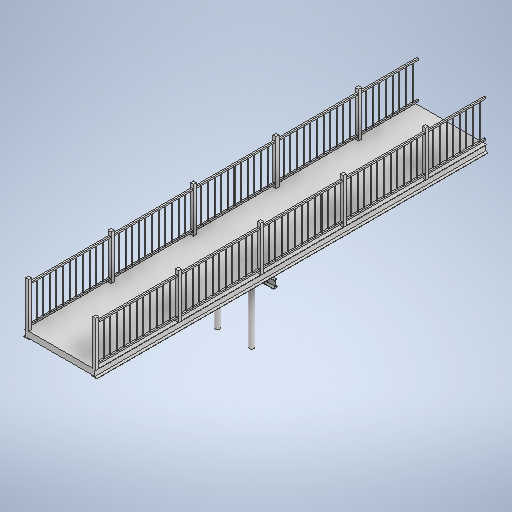
# Autodesk Inventor part: Bridge for Jude
Saved by Autodesk Inventor 2025 (Build 290162000, 162)
## iProperties
Created: 2024-06-25
Part Number: Bridge for Jude
Material: Generic
Document SubType Name: Modeling
Designer: track
Density: 1 g/cm^3
Appearance: Default
Author: track
Autodesk Inventor part; units mm, degrees
ref_plane "YZ Plane" through (0, 0, 0) normal (1, 0, 0) x (0, 1, 0)
ref_plane "XZ Plane" through (0, 0, 0) normal (0, 1, 0) x (-1, 0, 0)
ref_plane "XY Plane" through (0, 0, 0) normal (0, 0, 1) x (1, 0, 0)
sketch "Sketch4" plane through (0, 0, 0) normal (0, 0, 1) x (1, 0, 0)
  line L0 (838.2, -76.2) -> (-838.2, -76.2)
  line L1 (-838.2, -76.2) -> (-838.2, 76.2)
  line L2 (-838.2, 76.2) -> (838.2, 76.2)
  line L3 (838.2, 76.2) -> (838.2, -76.2)
  line L4 (838.2, -76.2) -> (-838.2, 76.2) construction
  line L5 (-838.2, -76.2) -> (838.2, 76.2) construction
  point P0 (0, 0)
  dimension "d8" = 1676.4
  dimension "d9" = 152.4
  constraints: 12 end point, 2 midpoint, 2 parallel, 1 horizontal, 1 perpendicular
  measures "d8" distance of L1.end L2.end
  measures "d9" distance of L0.end L1.end
extrude "Extrusion2" add sketch "Sketch4" against normal blind 9753.6
sketch "Sketch5" plane through (0, 0, 0) normal (0, 0, 1) x (1, 0, 0)
  line L0 (787.4, -101.6) -> (914.4, -101.6)
  line L1 (863.6, -76.2) -> (863.6, 50.8)
  line L2 (838.2, -76.2) -> (838.2, 50.8)
  line L3 (-838.2, 76.2) -> (838.2, 76.2) projected
  line L4 (889, 76.2) -> (812.8, 76.2)
  line L5 (-838.2, -76.2) -> (838.2, -76.2) projected
  line L6 (787.4, -101.6) -> (787.4, -95.25)
  line L7 (787.4, -95.25) -> (838.2, -76.2)
  line L8 (914.4, -101.6) -> (914.4, -95.25)
  line L9 (914.4, -95.25) -> (863.6, -76.2)
  line L10 (889, 76.2) -> (889, 66.675)
  line L11 (889, 66.675) -> (863.6, 50.8)
  line L12 (838.2, -76.2) -> (838.2, 76.2) projected
  line L13 (850.9, -101.6) -> (850.9, -34.364)
  line L14 (838.2, 50.8) -> (863.6, 50.8)
  line L15 (0, -76.2) -> (0, 76.2)
  line L16 (-787.4, -101.6) -> (-914.4, -101.6)
  line L17 (-863.6, -76.2) -> (-863.6, 50.8)
  line L18 (-838.2, -76.2) -> (-838.2, 50.8)
  line L19 (-889, 76.2) -> (-812.8, 76.2)
  line L20 (-787.4, -101.6) -> (-787.4, -95.25)
  line L21 (-787.4, -95.25) -> (-838.2, -76.2)
  line L22 (-914.4, -95.25) -> (-863.6, -76.2)
  line L23 (-889, 76.2) -> (-889, 66.675)
  line L24 (-889, 66.675) -> (-863.6, 50.8)
  line L25 (-787.4, -101.6) -> (-787.4, -95.25)
  line L26 (-914.4, -101.6) -> (-914.4, -95.25)
  line L27 (838.2, 50.8) -> (812.8, 66.675)
  line L28 (812.8, 66.675) -> (812.8, 76.2)
  line L29 (-838.2, 50.8) -> (-812.8, 66.675)
  line L30 (-812.8, 66.675) -> (-812.8, 76.2)
  point P0 (0, 0)
  dimension "d13" = 127
  dimension "d15" = 127
  dimension "d17" = 25.4
  dimension "d18" = 50.8
  dimension "d19" = 50.8
  dimension "d20" = 25.4
  dimension "d21" = 6.35
  dimension "d22" = 6.35
  dimension "d25" = 25.4
  dimension "d26" = 15.875
  dimension "d27" = 15.875
  constraints: 56 end point, 11 symmetric about line, 6 vertical, 3 midpoint, 2 collinear, 2 horizontal, 1 point on line, 1 other
  measures "d13" distance of L0.start L0.end
  measures "d15" distance of L1.start L1.end
  measures "d17" distance from line of L5 L0.start
  measures "d18" horizontal distance of L2.start L0.start
  measures "d19" horizontal distance of L1.start L0.end
  measures "d20" vertical distance of L0.end L1.start
  measures "d21" distance of L0.end L8.end
  measures "d22" distance of L0.start L6.end
  measures "d25" horizontal distance of L1.end L10.end
  measures "d26" vertical distance of L10.end L1.end
  measures "d27" vertical distance of L2.end L27.end
extrude "Extrusion3" add sketch "Sketch5" against normal blind 9753.6 contours L6 L7 L2 L14 L1 L9 L8 L0 | L12 L4 L10 L11 L14 | L21 L20 L16 L26 L22 L17 L24 L23 L19 L3 L30 L29 L18
sketch "Sketch6" plane through (-838.2, -76.2, 0) normal (0, -1, 0) x (1, 0, 0)
  line L0 (1676.4, 0) -> (1676.4, -9753.6) projected
  line L1 (0, 0) -> (0, -9753.6) projected
  line L2 (1676.4, -381) -> (0, -381)
  line L3 (0, -381) -> (0, -482.6)
  line L4 (0, -482.6) -> (1676.4, -482.6)
  line L5 (1676.4, -482.6) -> (1676.4, -381)
  line L6 (0, 0) -> (1676.4, 0) projected
  line L7 (1676.4, -1651) -> (0, -1651)
  line L8 (0, -1651) -> (0, -1752.6)
  line L9 (0, -1752.6) -> (1676.4, -1752.6)
  line L10 (1676.4, -1752.6) -> (1676.4, -1651)
  line L11 (1676.4, -2717.8) -> (0, -2717.8)
  line L12 (0, -2717.8) -> (0, -2819.4)
  line L13 (0, -2819.4) -> (1676.4, -2819.4)
  line L14 (1676.4, -2819.4) -> (1676.4, -2717.8)
  line L15 (1676.4, -3778.25) -> (0, -3778.25)
  line L16 (0, -3778.25) -> (0, -3879.85)
  line L17 (0, -3879.85) -> (1676.4, -3879.85)
  line L18 (1676.4, -3879.85) -> (1676.4, -3778.25)
  line L19 (1676.4, -4841.875) -> (0, -4841.875)
  line L20 (0, -4841.875) -> (0, -4943.475)
  line L21 (0, -4943.475) -> (1676.4, -4943.475)
  line L22 (1676.4, -4943.475) -> (1676.4, -4841.875)
  line L23 (1676.4, -6102.35) -> (0, -6102.35)
  line L24 (0, -6102.35) -> (0, -6203.95)
  line L25 (0, -6203.95) -> (1676.4, -6203.95)
  line L26 (1676.4, -6203.95) -> (1676.4, -6102.35)
  line L27 (1676.4, -7162.8) -> (0, -7162.8)
  line L28 (0, -7162.8) -> (0, -7264.4)
  line L29 (0, -7264.4) -> (1676.4, -7264.4)
  line L30 (1676.4, -7264.4) -> (1676.4, -7162.8)
  line L31 (1676.4, -8331.2) -> (0, -8331.2)
  line L32 (0, -8331.2) -> (0, -8229.6)
  line L33 (0, -8229.6) -> (1676.4, -8229.6)
  line L34 (1676.4, -8229.6) -> (1676.4, -8331.2)
  line L35 (1676.4, -9474.2) -> (0, -9474.2)
  line L36 (0, -9474.2) -> (0, -9575.8)
  line L37 (0, -9575.8) -> (1676.4, -9575.8)
  line L38 (1676.4, -9575.8) -> (1676.4, -9474.2)
  line L39 (1676.4, -9753.6) -> (0, -9753.6) projected
  point P0 (0, -9474.2)
  point P1 (0, -8331.2)
  point P2 (0, -7162.8)
  point P3 (0, -6102.35)
  point P4 (0, -4841.875)
  point P5 (0, -3778.25)
  point P6 (0, -2717.8)
  point P7 (0, -1651)
  point P8 (0, -381)
  dimension "d31" = 101.6
  dimension "d32" = 381
  dimension "d34" = 101.6
  dimension "d35" = 1168.4
  dimension "d36" = 101.6
  dimension "d37" = 101.6
  dimension "d38" = 965.2
  dimension "d39" = 958.85
  dimension "d40" = 101.6
  dimension "d41" = 962.025
  dimension "d42" = 1158.875
  dimension "d43" = 101.6
  dimension "d44" = 958.85
  dimension "d45" = 101.6
  dimension "d46" = 965.2
  dimension "d47" = 177.8
  dimension "d48" = 101.6
  dimension "d49" = 101.6
  constraints: 72 end point, 18 parallel, 9 horizontal, 9 perpendicular, 20 other
  measures "d31" distance between parallel lines of L2 L4
  measures "d32" distance between parallel lines of L6 L2
  measures "d34" distance between parallel lines of L7 L9
  measures "d35" distance between parallel lines of L7 L4
  measures "d36" distance between parallel lines of L13 L11
  measures "d37" distance between parallel lines of L17 L15
  measures "d38" distance between parallel lines of L9 L11
  measures "d39" distance between parallel lines of L13 L15
  measures "d40" distance between parallel lines of L21 L19
  measures "d41" distance between parallel lines of L17 L19
  measures "d42" distance between parallel lines of L21 L23
  measures "d43" distance between parallel lines of L25 L23
  measures "d44" distance between parallel lines of L25 L27
  measures "d45" distance between parallel lines of L29 L27
  measures "d46" distance between parallel lines of L29 L33
  measures "d47" distance between parallel lines of L39 L37
  measures "d48" distance between parallel lines of L37 L35
  measures "d49" distance between parallel lines of L31 L33
extrude "Extrusion4" add sketch "Sketch6" along normal blind 25.4 contours L0 L4 L1 L2 | L0 L9 L1 L7 | L0 L13 L1 L11 | L0 L17 L1 L15 | L0 L21 L1 L19 | L0 L25 L1 L23 | L0 L29 L1 L27 | L0 L31 L1 L33 | L0 L37 L1 L35
sketch "Sketch8" plane through (-863.6, 50.8, -9753.6) normal (-1, 0, 0) x (0, 0, 1)
  line L0 (0, 0) -> (0, -127) projected
  line L1 (9753.6, 0) -> (9753.6, -127) projected
  line L2 (9753.6, -152.4) -> (0, -152.4) projected
  line L3 (5410.2, -152.4) -> (5410.2, -165.1)
  line L4 (5410.2, -165.1) -> (5384.8, -171.45)
  line L5 (5384.8, -171.45) -> (5384.8, -298.45)
  line L6 (5384.8, -298.45) -> (5435.6, -323.85)
  line L7 (5435.6, -323.85) -> (5435.6, -330.2)
  line L8 (5435.6, -330.2) -> (5321.3, -330.2)
  line L9 (5321.3, -330.2) -> (5321.3, -323.85)
  line L10 (5372.1, -298.45) -> (5372.1, -171.45)
  line L11 (5410.2, -152.4) -> (5346.7, -152.4)
  line L12 (5378.45, -325.0091) -> (5378.45, -152.4) construction
  line L13 (5372.1, -171.45) -> (5346.7, -165.1)
  line L14 (5346.7, -165.1) -> (5346.7, -152.4)
  line L15 (5372.1, -298.45) -> (5384.8, -298.45) construction
  line L16 (5321.3, -323.85) -> (5372.1, -298.45)
  point P0 (9753.6, -50.8)
  point P1 (9753.6, -63.5)
  dimension "d61" = 12.7
  dimension "d62" = 6.35
  dimension "d63" = 6.35
  dimension "d64" = 6.35
  dimension "d65" = 50.8
  dimension "d66" = 25.4
  dimension "d67" = 25.4
  dimension "d68" = 25.4
  dimension "d69" = 6.35
  dimension "d70" = 50.8
  dimension "d71" = 90
  dimension "d73" = 127
  dimension "d74" = 177.8
  dimension "d75" = 127
  dimension "d76" = 6.35
  dimension "d77" = 4368.8
  constraints: 26 end point, 5 vertical, 3 parallel, 2 midpoint, 2 point on line, 1 collinear, 3 other
  measures "d61" distance between parallel lines of L10 L5
  measures "d62" distance between parallel lines of L5 L12
  measures "d63" vertical distance of L4.end L3.end
  measures "d64" distance of L6.end L7.end
  measures "d65" horizontal distance of L5.end L6.end
  measures "d66" vertical distance of L5.end L6.end
  measures "d67" horizontal distance of L3.end L4.end
  measures "d68" horizontal distance of L10.end L13.end
  measures "d69" distance of L9.start L9.end
  measures "d70" horizontal distance of L9.end L10.start
  measures "d71" angle of L15 L10
  measures "d73" distance of L4.end L5.end
  measures "d75" distance of L10.start L10.end
  measures "d76" vertical distance of L10.end L13.end
  measures "d77" distance from line of point (9753.6, -63.5) L5
extrude "Extrusion5" add sketch "Sketch8" along normal blind 120.65 and the other way blind 1866.9
sketch "Sketch9" plane through (-984.25, -279.4, -4318) normal (0, -1, 0) x (1, 0, 0)
  line L0 (0, -25.4) -> (0, -88.9) projected
  line L1 (0, -57.15) -> (1266.7426, -57.15)
  circle A0 centre (533.4, -57.15) radius 57.15
  circle A1 centre (1384.3, -57.15) radius 57.15
  point P0 (984.25, 4318)
  dimension "d82" = 114.3
  dimension "d83" = 533.4
  dimension "d84" = 114.3
  dimension "d85" = 850.9
  constraints: 2 centre point, 2 end point, 2 point on line, 1 horizontal, 1 midpoint
  measures "d82" diameter of A0
  measures "d83" distance from line of L0 A0.centre
  measures "d84" diameter of A1
  measures "d85" distance of A0.centre A1.centre
extrude "Extrusion6" add sketch "Sketch9" along normal blind 1587.5
sketch "Sketch10" plane through (-889, 76.2, 0) normal (0, 1, 0) x (1, 0, 0)
  line L0 (1778, 0) -> (1778, 9753.6) projected
  line L1 (1778, 0) -> (1701.8, 0)
  line L2 (1701.8, 0) -> (1701.8, 76.2)
  line L3 (1701.8, 76.2) -> (1778, 76.2)
  line L4 (1778, 76.2) -> (1778, 0)
  line L5 (889, 0) -> (889, 9753.6) construction
  line L6 (0, 9753.6) -> (1778, 9753.6) projected
  point P0 (0, 0)
  dimension "d88" = 76.2
  dimension "d89" = 76.2
  constraints: 10 end point, 2 parallel, 1 horizontal, 1 midpoint, 1 perpendicular
  measures "d88" distance of L2.end L3.end
  measures "d89" distance of L1.end L2.end
extrude "Extrusion7" add sketch "Sketch10" along normal blind 1117.6
sketch "Sketch11" plane through (889, 76.2, -76.2) normal (0, 0, -1) x (-1, 0, 0)
  line L0 (19.05, 114.3) -> (57.15, 114.3)
  line L1 (57.15, 114.3) -> (57.15, 76.2)
  line L2 (57.15, 76.2) -> (19.05, 76.2)
  line L3 (19.05, 76.2) -> (19.05, 114.3)
  line L4 (19.05, 114.3) -> (57.15, 76.2) construction
  line L5 (57.15, 114.3) -> (19.05, 76.2) construction
  line L6 (19.05, 1016) -> (57.15, 1016)
  line L7 (57.15, 1016) -> (57.15, 977.9)
  line L8 (57.15, 977.9) -> (19.05, 977.9)
  line L9 (19.05, 977.9) -> (19.05, 1016)
  line L10 (19.05, 1016) -> (57.15, 977.9) construction
  line L11 (57.15, 1016) -> (19.05, 977.9) construction
  line L12 (76.2, 0) -> (76.2, 1117.6) projected
  line L13 (1778, 0) -> (0, 0) projected
  point P0 (889, -76.2)
  point P1 (38.1, 95.25)
  point P2 (38.1, 996.95)
  dimension "d92" = 38.1
  dimension "d93" = 38.1
  dimension "d94" = 38.1
  dimension "d95" = 76.2
  dimension "d96" = 863.6
  dimension "d97" = 38.1
  dimension "d98" = 38.1
  constraints: 24 end point, 4 midpoint, 4 parallel, 2 horizontal, 2 perpendicular, 1 point on line
  measures "d92" distance of L0.end L1.end
  measures "d93" distance of L0.start L0.end
  measures "d94" distance from line of L12 point (38.1, 95.25)
  measures "d95" distance between parallel lines of L13 L2
  measures "d96" distance between parallel lines of L8 L0
  measures "d97" distance of L6.end L7.end
  measures "d98" distance of L6.start L6.end
extrude "Extrusion8" add sketch "Sketch11" along normal blind 1981.2
sketch "Sketch12" plane through (869.95, 190.5, -76.2) normal (0, 1, 0) x (1, 0, 0)
  line L0 (-38.1, 0) -> (0, 0) projected
  line L1 (-19.05, 0) -> (-19.05, 1981.2) construction
  line L2 (0, 1981.2) -> (-38.1, 1981.2) projected
  line L3 (-12.7, 152.4) -> (-25.4, 152.4)
  line L4 (-25.4, 152.4) -> (-25.4, 165.1)
  line L5 (-25.4, 165.1) -> (-12.7, 165.1)
  line L6 (-12.7, 165.1) -> (-12.7, 152.4)
  line L7 (-12.7, 152.4) -> (-25.4, 165.1) construction
  line L8 (-25.4, 152.4) -> (-12.7, 165.1) construction
  line L9 (-25.4, 317.5) -> (-25.4, 330.2)
  line L10 (-25.4, 330.2) -> (-12.7, 330.2)
  line L11 (-12.7, 330.2) -> (-12.7, 317.5)
  line L12 (-12.7, 317.5) -> (-25.4, 317.5)
  line L13 (-25.4, 482.6) -> (-25.4, 495.3)
  line L14 (-25.4, 495.3) -> (-12.7, 495.3)
  line L15 (-12.7, 495.3) -> (-12.7, 482.6)
  line L16 (-12.7, 482.6) -> (-25.4, 482.6)
  line L17 (-25.4, 647.7) -> (-25.4, 660.4)
  line L18 (-25.4, 660.4) -> (-12.7, 660.4)
  line L19 (-12.7, 660.4) -> (-12.7, 647.7)
  line L20 (-12.7, 647.7) -> (-25.4, 647.7)
  line L21 (-25.4, 812.8) -> (-25.4, 825.5)
  line L22 (-25.4, 825.5) -> (-12.7, 825.5)
  line L23 (-12.7, 825.5) -> (-12.7, 812.8)
  line L24 (-12.7, 812.8) -> (-25.4, 812.8)
  line L25 (-25.4, 977.9) -> (-25.4, 990.6)
  line L26 (-25.4, 990.6) -> (-12.7, 990.6)
  line L27 (-12.7, 990.6) -> (-12.7, 977.9)
  line L28 (-12.7, 977.9) -> (-25.4, 977.9)
  line L29 (-25.4, 1143) -> (-25.4, 1155.7)
  line L30 (-25.4, 1155.7) -> (-12.7, 1155.7)
  line L31 (-12.7, 1155.7) -> (-12.7, 1143)
  line L32 (-12.7, 1143) -> (-25.4, 1143)
  line L33 (-25.4, 1308.1) -> (-25.4, 1320.8)
  line L34 (-25.4, 1320.8) -> (-12.7, 1320.8)
  line L35 (-12.7, 1320.8) -> (-12.7, 1308.1)
  line L36 (-12.7, 1308.1) -> (-25.4, 1308.1)
  line L37 (-25.4, 1473.2) -> (-25.4, 1485.9)
  line L38 (-25.4, 1485.9) -> (-12.7, 1485.9)
  line L39 (-12.7, 1485.9) -> (-12.7, 1473.2)
  line L40 (-12.7, 1473.2) -> (-25.4, 1473.2)
  line L41 (-25.4, 1638.3) -> (-25.4, 1651)
  line L42 (-25.4, 1651) -> (-12.7, 1651)
  line L43 (-12.7, 1651) -> (-12.7, 1638.3)
  line L44 (-12.7, 1638.3) -> (-25.4, 1638.3)
  line L45 (-25.4, 1803.4) -> (-25.4, 1816.1)
  line L46 (-25.4, 1816.1) -> (-12.7, 1816.1)
  line L47 (-12.7, 1816.1) -> (-12.7, 1803.4)
  line L48 (-12.7, 1803.4) -> (-25.4, 1803.4)
  point P0 (-869.95, -76.2)
  point P1 (-19.05, 158.75)
  dimension "d101" = 12.7
  dimension "d102" = 12.7
  dimension "d103" = 152.4
  dimension "d106" = 165.1
  constraints: 94 end point, 4 midpoint, 2 parallel, 1 horizontal, 1 perpendicular, 1 point on line, 1 vertical, 80 other
  measures "d101" distance of L3.start L3.end
  measures "d102" distance of L5.end L3.start
  measures "d103" distance between parallel lines of L0 L3
  measures "d106" distance of L3.end L9.start
extrude "Extrusion9" add sketch "Sketch12" along normal blind 863.6
pattern_linear "Rectangular Pattern1" count 2 spacing 1676.4 along (-1, 0, 0) count 5 spacing 2057.4 along (0, 0, -1) of "Extrusion9", "Extrusion8", "Extrusion7"
sketch "Sketch13" plane through (-787.4, -101.6, -4841.875) normal (0, -1, 0) x (1, 0, 0)
  line L0 (-57.15, -5445.125) -> (-19.05, -5445.125) projected
  line L1 (1701.8, -4911.725) -> (-57.15, -4911.725)
  line L2 (-57.15, -4911.725) -> (-57.15, -5445.125)
  line L3 (-57.15, -5445.125) -> (1701.8, -5445.125)
  line L4 (1701.8, -5445.125) -> (1701.8, -4911.725)
  point P0 (787.4, 4841.875)
  constraints: 8 end point, 2 parallel, 1 horizontal, 1 perpendicular
extrude "Extrusion10" cut sketch "Sketch13" against normal up to surface (1193.8 mm away)
body "Solid2"
